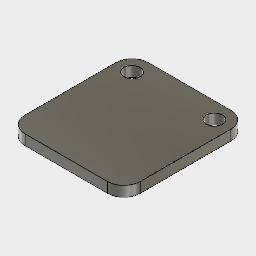
3006 MAX98357 (Autodesk Fusion 360 design; units mm, degrees)
Autodesk Fusion 360 part; units mm, degrees
sketch "Sketch1" plane through (0, 0, 0) normal (0, 0, 1) x (1, 0, 0)
  line L0 (0, 0) -> (17.78, 0)
  line L1 (17.78, 0) -> (17.78, 19.05)
  line L2 (17.78, 19.05) -> (0, 19.05)
  line L3 (0, 19.05) -> (0, 0)
  circle A0 centre (2.54, 16.51) radius 1.25
  line L4 (8.89, 19.05) -> (8.89, 0) construction
  line L5 (0, 9.525) -> (17.78, 9.525) construction
  circle A1 centre (15.24, 16.51) radius 1.25
  dimension "d1" = 17.78
  dimension "d2" = 19.05
  dimension "d3" = 2.5
  dimension "d4" = 16.51
  dimension "d5" = 2.54
  measures "d1" distance of L0.start L0.end
  measures "d2" distance of L0.start L2.end
  measures "d3" diameter of A0
  measures "d4" distance of L0 A0.centre
  measures "d5" distance of L3 A0.centre
extrude "Extrude1" add sketch "Sketch1" along normal blind 1.6
fillet "Fillet1" radius 2.54 4 edges at (17.78, 0, 0.8) (0, 0, 0.8) (0, 19.05, 0.8) (17.78, 19.05, 0.8)
